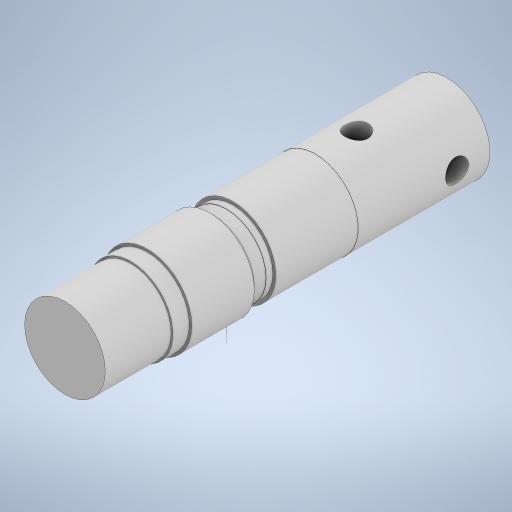
# Autodesk Inventor part: Mangon_Conducido
Saved by Autodesk Inventor 2024 (Build 280153000, 153)
## iProperties
Created: 2026-01-05
Part Number: Mangon_Conducido
Material: Generic
Document SubType Name: Modeling
Designer: eduso
Density: 1 g/cm^3
Appearance: Default
Cido_Testero_007: 4,000 mm
Cido_Espacio_008: 50,000 mm
Cido_Inteerior_Tubo_009: 80,000 mm
Author: eduso
Autodesk Inventor part; units mm, degrees
ref_plane "YZ Plane" through (0, 0, 0) normal (1, 0, 0) x (0, 1, 0)
ref_plane "XY Plane" through (0, 0, 0) normal (0, 0, 1) x (1, 0, 0)
sketch "Sketch1" plane through (0, 0, 0) normal (0, 1, 0) x (-1, 0, 0)
  line L0 (24, 8) -> (27, 8)
  line L1 (27, 8) -> (27, 48)
  line L2 (27, 48) -> (25.5, 48)
  line L3 (25.5, 48) -> (25.5, 58)
  line L4 (26, 208) -> (25, 208)
  line L5 (25, 248) -> (25, 248)
  line L6 (0, 138) -> (0, -122.7414) construction
  line L7 (24, 8) -> (24, 0)
  line L8 (0, 98) -> (0, 0)
  line L9 (24, 0) -> (24.2, 0)
  line L10 (24.2, 0) -> (24.2, -4)
  line L11 (24.2, -4) -> (26, -4)
  line L12 (26, -4) -> (26, -54)
  line L13 (26, -54) -> (26.1, -54)
  line L14 (26.1, -54) -> (26.1, -134)
  line L15 (26.1, -134) -> (0, -134)
  line L16 (0, 0) -> (0, -134)
  line L17 (24, 0) -> (24.2, 0)
  line L18 (25.5, 58) -> (24.5, 58)
  line L19 (24.5, 58) -> (24.5, 98)
  line L20 (24.5, 98) -> (0, 98)
  dimension "d2" = 40
  dimension "d4" = 8
  dimension "d16" = 10
  dimension "d71" = 27
  dimension "d78" = 24
  dimension "d82" = 4
  dimension "d83" = 50
  dimension "d84" = 24.2
  dimension "d85" = 26.1
  dimension "d86" = 80
  dimension "d88" = 25.5
  dimension "d89" = 26
  dimension "d90" = 40
  dimension "d92" = 24.5
  constraints: 42 end point, 8 perpendicular, 4 horizontal, 3 vertical, 2 collinear, 2 point on line, 3 other
  measures "d2" distance of L0.end L1.end
  measures "d4" distance of L0.start L7.end
  measures "d16" distance of L2.end L3.end
  measures "d71" distance between parallel lines of L1 L8
  measures "d78" distance between parallel lines of L6 L7
  measures "d82" distance of L9.end L10.end
  measures "d83" distance of L11.end L12.end
  measures "d84" distance between parallel lines of L6 L10
  measures "d85" distance between parallel lines of L16 L14
  measures "d86" distance of L13.end L14.end
  measures "d88" distance between parallel lines of L6 L3
  measures "d89" distance between parallel lines of L6 L12
  measures "d90" distance of L18.end L19.end
  measures "d92" distance between parallel lines of L8 L19
ref_plane "Work Plane1" through (0, 15, 0) normal (0, 1, 0) x (-1, 0, 0)
sketch "Sketch3" plane through (0, 15, 0) normal (0, 1, 0) x (-1, 0, 0)
  circle A0 centre (0, -79) radius 7
  point P0 (0, 0)
  dimension "d22" = 14
  dimension "d66" = 79
  constraints: 1 centre point
  measures "d22" diameter of A0
  measures "d66" distance of point (0, 0) A0.centre
sketch "Sketch4" plane through (0, 0, 0) normal (1, 0, 0) x (0, 1, 0)
  circle A0 centre (0, -114) radius 7
  point P0 (0, 0)
  dimension "d28" = 14
  dimension "d67" = 114
  constraints: 1 centre point
  measures "d28" diameter of A0
  measures "d67" distance of point (0, 0) A0.centre
revolve "Revolution1" add sketch "Sketch1" angle 360 about axis through (0, 0, 98) along (0, 0, -1)
extrude "Extrusion5" cut sketch "Sketch3" along normal blind 20 and the other way blind 45
extrude "Extrusion6" cut sketch "Sketch4" along normal blind 35 and the other way blind 30
chamfer "Chamfer3" distance 2 angle 45 1 edges at (27, 0, 8)
sketch "Sketch5" plane through (0, 0, 0) normal (0, 1, 0) x (-1, 0, 0)
  line L0 (24, 8) -> (24, 0) projected
  point P0 (0, 0)
sketch "Sketch6" plane through (0, 0, 0) normal (1, 0, 0) x (0, 1, 0)
  line L0 (0, 0) -> (-46.2751, 0) construction
  constraints: 2 end point, 1 horizontal
equation "\"DiametroInterior\" = 52.2"
body "Solid4"
